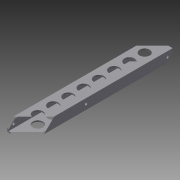
# Autodesk Inventor part: 2x1 mounting
Saved by Autodesk Inventor 2015 (Build 190159000, 159)
## iProperties
Created: 2015-02-22
Part Number: 2x1 mounting
Material: Generic
Document SubType Name: Modeling
Designer: Jarod
Density: 1 g/cm^3
Appearance: Default
Author: Jarod
Autodesk Inventor part; units mm, degrees
ref_plane "YZ Plane" through (0, 0, 0) normal (1, 0, 0) x (0, 1, 0)
ref_plane "XZ Plane" through (0, 0, 0) normal (0, 1, 0) x (-1, 0, 0)
ref_plane "XY Plane" through (0, 0, 0) normal (0, 0, 1) x (1, 0, 0)
sketch "Sketch1" plane through (0, 0, 0) normal (0, 0, 1) x (1, 0, 0)
  line L0 (0, 0) -> (50.8, 0)
  line L1 (50.8, 0) -> (50.8, 25.4)
  line L2 (50.8, 25.4) -> (0, 25.4)
  line L3 (0, 25.4) -> (0, 0)
  line L4 (3.175, 3.175) -> (47.625, 3.175)
  line L5 (47.625, 3.175) -> (47.625, 22.225)
  line L6 (47.625, 22.225) -> (3.175, 22.225)
  line L7 (3.175, 22.225) -> (3.175, 3.175)
  dimension "d0" = 50.8
  dimension "d1" = 25.4
  dimension "d2" = 44.45
  dimension "d3" = 19.05
  dimension "d4" = 3.175
  dimension "d5" = 3.175
  constraints: 16 end point, 4 parallel, 2 horizontal, 2 perpendicular
  measures "d0" distance of L2.end L1.end
  measures "d1" distance of L1.end L0.end
  measures "d2" distance of L6.end L5.end
  measures "d3" distance of L5.end L4.end
  measures "d4" distance between parallel lines of L3 L7
  measures "d5" distance between parallel lines of L0 L4
extrude "Extrusion1" add sketch "Sketch1" against normal blind 361.95
sketch "Sketch2" plane through (50.8, 0, 0) normal (1, 0, 0) x (0, 0, -1)
  line L0 (0, 0) -> (0, 25.4) projected
  line L1 (0, 0) -> (361.95, 0) projected
  line L2 (361.95, 25.4) -> (361.95, 0) projected
  line L3 (0, 25.4) -> (361.95, 25.4) projected
  point P0 (146.05, 12.7)
  point P1 (349.25, 12.7)
  dimension "d8" = 12.7
  dimension "d9" = 12.7
  dimension "d10" = 215.9
  dimension "d11" = 12.7
  measures "d8" distance from line of L2 point (349.25, 12.7)
  measures "d9" distance from line of L3 point (349.25, 12.7)
  measures "d10" distance from line of point (146.05, 12.7) L2
  measures "d11" distance from line of L3 point (146.05, 12.7)
hole "Hole1" at (50.8, 12.7, -146.05) at (50.8, 12.7, -349.25) direction (-1, 0, 0) diameter 6.35 end through all
sketch "Sketch3" plane through (50.8, 0, 0) normal (1, 0, 0) x (0, 0, -1)
  circle A0 centre (146.05, 12.7) radius 3.175 projected
  circle A1 centre (349.25, 12.7) radius 3.175 projected
  line L0 (0, 0) -> (0, 25.4) projected
  line L1 (0, 0) -> (361.95, 0) projected
  line L2 (361.95, 25.4) -> (361.95, 0) projected
  line L3 (0, 25.4) -> (361.95, 25.4) projected
  point P0 (12.7, 12.7)
  dimension "d19" = 12.7
  dimension "d20" = 12.7
  measures "d19" distance from line of L3 point (12.7, 12.7)
  measures "d20" distance from line of L0 point (12.7, 12.7)
hole "Hole2" at (50.8, 12.7, -12.7) direction (-1, 0, 0) diameter 6.35 end through all
sketch "Sketch4" plane through (0, 25.4, 0) normal (0, 1, 0) x (1, 0, 0)
  line L0 (50.8, 0) -> (0, 0) projected
  line L1 (50.8, 0) -> (50.8, 361.95) projected
  line L2 (0, 361.95) -> (50.8, 361.95) projected
  line L3 (0, 0) -> (0, 361.95) projected
  point P0 (25.4, 50.8)
  dimension "d28" = 25.4
  dimension "d29" = 50.8
  measures "d28" distance from line of L3 point (25.4, 50.8)
  measures "d29" distance from line of L0 point (25.4, 50.8)
hole "Hole3" at (25.4, 25.4, -50.8) direction (0, -1, 0) diameter 25.4 end through all
pattern_linear "Rectangular Pattern1" count 8 spacing 38.1 along (0, 0, -1) of "Hole3"
body "Solid1"
